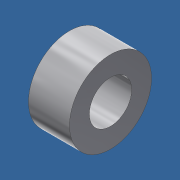
# Autodesk Inventor part: BN5281_3.1x6x3
Saved by Autodesk Inventor 2021 (Build 250183000, 183)
## iProperties
Created: 2020-11-25
Part Number: BN5281_3.1x6x3
Material: PA6.6
Description: Douilles d'écartement
Document SubType Name: Modeling
Designer: Jean-Marc.VULLIAMY
Authority: BN5281
Density: 1.14 g/cm^3
Appearance: Lisse - Blanc
Material number: ---
Author: Jean-Marc.VULLIAMY
Autodesk Inventor part; units mm, degrees
ref_plane "Plan YZ" through (0, 0, 0) normal (1, 0, 0) x (0, 1, 0)
ref_plane "Plan XZ" through (0, 0, 0) normal (0, 1, 0) x (-1, 0, 0)
ref_plane "Plan XY" through (0, 0, 0) normal (0, 0, 1) x (1, 0, 0)
sketch "Esquisse1" plane through (0, 0, 0) normal (0, 0, 1) x (1, 0, 0)
  line L0 (0, 3) -> (3, 3)
  line L1 (3, 3) -> (3, 1.55)
  line L2 (3, 1.55) -> (0, 1.55)
  line L3 (0, 1.55) -> (0, 3)
  line L4 (-0.6, 0) -> (3.6, 0) construction
  point P0 (0, 0)
  dimension "d0" = 3.1
  dimension "d1" = 6
  dimension "d2" = 3
  constraints: 8 end point, 2 parallel, 1 horizontal, 1 perpendicular, 1 point on line
  measures "d0" diameter of L2 L4
  measures "d1" diameter of L0 L4
  measures "d2" distance of L0.start L0.end
revolve "Révolution1" add sketch "Esquisse1" angle 360 about axis through (-10, 0, 0) along (1, 0, 0)
